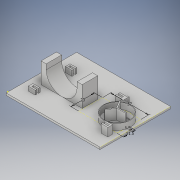
# Autodesk Inventor part: base
Saved by Autodesk Inventor 2019 (Build 230136000, 136)
## iProperties
Created: 2022-02-03
Part Number: base
Material: Generic
Document SubType Name: Modeling
Designer: josec
Density: 1 g/cm^3
Appearance: Default
Author: josec
Autodesk Inventor part; units mm, degrees
ref_plane "YZ Plane" through (0, 0, 0) normal (1, 0, 0) x (0, 1, 0)
ref_plane "XZ Plane" through (0, 0, 0) normal (0, 1, 0) x (-1, 0, 0)
ref_plane "XY Plane" through (0, 0, 0) normal (0, 0, 1) x (1, 0, 0)
sketch "Sketch1" plane through (0, 0, 0) normal (0, 1, 0) x (-1, 0, 0)
  line L0 (0, 0) -> (-90, 0)
  line L1 (-90, 0) -> (-90, -60)
  line L2 (-90, -60) -> (0, -60)
  line L3 (0, -60) -> (0, 0)
  dimension "d0" = 90
  dimension "d1" = 60
  constraints: 8 end point, 2 parallel, 1 horizontal, 1 perpendicular
  measures "d0" distance of L2.end L1.end
  measures "d1" distance of L1.end L0.end
extrude "Extrusion1" add sketch "Sketch1" along normal blind 2
sketch "Sketch2" plane through (0, 2, 0) normal (0, 1, 0) x (1, 0, 0)
  line L0 (90, 0) -> (90, 60) construction
  line L1 (90, 60) -> (85, 60) construction
  line L2 (90, 60) -> (0, 60) construction
  line L3 (85, 60) -> (85, 0) construction
  line L4 (0, 0) -> (90, 0) construction
  line L5 (85, 30) -> (85, 35.5) construction
  line L6 (85, 35.5) -> (85, 30) construction
  line L7 (85, 30) -> (85, 24.5) construction
  line L8 (85, 24.5) -> (79, 24.5)
  line L9 (79, 24.5) -> (79, 23.5)
  line L10 (79, 23.5) -> (85, 23.5)
  line L11 (85, 23.5) -> (85, 24.5)
  line L12 (85, 35.5) -> (79, 35.5)
  line L13 (79, 35.5) -> (79, 36.5)
  line L14 (79, 36.5) -> (85, 36.5)
  line L15 (85, 36.5) -> (85, 35.5)
  dimension "d4" = 5
  dimension "d5" = 5.5
  dimension "d6" = 5.5
  dimension "d7" = 6
  dimension "d8" = 1
  dimension "d9" = 1
  constraints: 26 end point, 4 parallel, 4 point on line, 2 horizontal, 2 perpendicular, 1 collinear, 1 midpoint, 1 vertical
  measures "d4" distance of L0.end L1.end
  measures "d5" distance of L5.start L5.end
  measures "d6" distance of L5.start L7.end
  measures "d7" distance of L10.end L9.end
  measures "d8" distance of L9.end L8.end
  measures "d9" distance of L12.end L13.end
extrude "Extrusion2" cut sketch "Sketch2" against normal through all
sketch "Sketch3" plane through (0, 2, 0) normal (0, 1, 0) x (1, 0, 0)
  line L0 (85, 35.5) -> (79, 35.5) construction
  line L1 (85, 24.5) -> (79, 24.5) construction
  line L2 (79, 35.5) -> (79, 24.5) construction
  line L3 (79, 30) -> (72.5, 30) construction
  line L4 (72.5, 30) -> (72.5, 32.5) construction
  line L5 (72.5, 32.5) -> (67.5, 32.5) construction
  line L6 (67.5, 32.5) -> (67.5, 27.5) construction
  line L7 (67.5, 27.5) -> (72.5, 27.5) construction
  line L8 (72.5, 27.5) -> (72.5, 32.5) construction
  line L9 (67.5, 27.5) -> (70.5, 27.5) construction
  line L10 (67.5, 32.5) -> (70.5, 32.5) construction
  arc A0 (70.5, 27.5) -> (70.5, 32.5) centre (69.9375, 30) ccw
  line L11 (70.5, 32.5) -> (67.5, 32.5) construction
  line L12 (67.5, 32.5) -> (67.5, 27.5) construction
  line L13 (67.5, 32.5) -> (70.5, 32.5)
  line L14 (67.5, 32.5) -> (67.5, 27.5)
  line L15 (67.5, 27.5) -> (70.5, 27.5)
  point P0 (0, 0)
  dimension "d12" = 6.5
  dimension "d15" = 2.5
  dimension "d16" = 5
  dimension "d17" = 5
  dimension "d18" = 3
  dimension "d19" = 3
  constraints: 28 end point, 4 perpendicular, 3 point on circle, 2 collinear, 2 horizontal, 2 parallel, 2 point on line, 2 vertical, 1 centre point, 1 midpoint
  measures "d12" distance of L3.start L3.end
  measures "d15" distance of L3.end L4.end
  measures "d16" distance of L7.end L6.end
  measures "d17" distance of L6.end L5.end
  measures "d18" distance of L6.end L9.end
  measures "d19" distance of L5.end L10.end
extrude "Extrusion3" cut sketch "Sketch3" against normal through all
sketch "Sketch5" plane through (0, 2, 0) normal (0, 1, 0) x (1, 0, 0)
  line L0 (85, 35.5) -> (85, 36.5) construction
  line L1 (85, 36.5) -> (67.5, 36.5) construction
  line L2 (67.5, 36.5) -> (67.5, 23.5) construction
  line L3 (67.5, 23.5) -> (85, 23.5) construction
  line L4 (85, 23.5) -> (85, 36.5) construction
  circle A0 centre (76.25, 30) radius 12.5 construction
  line L5 (76.25, 30) -> (85, 30) construction
  line L6 (85, 30) -> (85, 30.5) construction
  line L7 (85, 30.5) -> (76.25, 30.5)
  line L8 (76.25, 30.5) -> (76.25, 29.5)
  line L9 (76.25, 29.5) -> (85, 29.5)
  line L10 (85, 29.5) -> (85, 30.5)
  line L11 (76.25, 30) -> (71.875, 37.5777) construction
  line L12 (71.875, 37.5777) -> (71.442, 37.3277) construction
  line L13 (71.442, 37.3277) -> (75.817, 29.75)
  line L14 (75.817, 29.75) -> (76.683, 30.25)
  line L15 (76.683, 30.25) -> (72.308, 37.8277)
  line L16 (72.308, 37.8277) -> (71.442, 37.3277)
  line L17 (76.25, 30) -> (71.875, 22.4223) construction
  line L18 (71.875, 22.4223) -> (72.308, 22.1723) construction
  line L19 (72.308, 22.1723) -> (76.683, 29.75)
  line L20 (76.683, 29.75) -> (75.817, 30.25)
  line L21 (75.817, 30.25) -> (71.442, 22.6723)
  line L22 (71.442, 22.6723) -> (72.308, 22.1723)
  point P0 (0, 0)
  dimension "d32" = 13
  dimension "d33" = 25
  dimension "d34" = 0.5
  dimension "d35" = 1
  dimension "d38" = 360
  constraints: 44 end point, 4 parallel, 2 coincident, 2 horizontal, 2 perpendicular, 1 centre point, 1 midpoint, 1 point on line, 35 other
  measures "d32" distance of L2.end L1.end
  measures "d33" diameter of A0
  measures "d34" distance of L5.end L6.end
  measures "d35" distance of L8.end L7.end
extrude "Extrusion4" add sketch "Sketch5" along normal blind 10
sketch "Sketch6" plane through (0, 2, 0) normal (0, 1, 0) x (1, 0, 0)
  line L0 (85, 36.5) -> (85, 35.5) construction
  line L1 (85, 36.5) -> (67.5, 36.5) construction
  line L2 (67.5, 36.5) -> (67.5, 23.5) construction
  line L3 (67.5, 23.5) -> (85, 23.5) construction
  line L4 (85, 23.5) -> (85, 36.5) construction
  circle A0 centre (76.25, 30) radius 12.5
  circle A1 centre (76.25, 30) radius 13
  point P0 (0, 0)
  dimension "d42" = 13
  dimension "d43" = 25
  dimension "d44" = 26
  constraints: 8 end point, 2 centre point, 2 parallel, 1 coincident, 1 horizontal, 1 perpendicular
  measures "d42" distance of L2.end L1.end
  measures "d43" diameter of A0
  measures "d44" diameter of A1
extrude "Extrusion5" add sketch "Sketch6" along normal blind 6
sketch "Sketch7" plane through (0, 2, 0) normal (0, 1, 0) x (1, 0, 0)
  line L0 (90, 0) -> (90, 60) construction
  line L1 (90, 30) -> (90, 14) construction
  line L2 (90, 14) -> (0, 14) construction
  line L3 (0, 60) -> (0, 0) construction
  line L4 (90, 14) -> (85, 14) construction
  line L5 (85, 14) -> (11, 14) construction
  line L6 (11, 14) -> (11, 12.4) construction
  line L7 (11, 12.4) -> (85, 12.4) construction
  line L8 (85, 12.4) -> (85, 14) construction
  line L9 (85, 14) -> (85, 12.4)
  line L10 (85, 12.4) -> (80, 12.4)
  line L11 (85, 14) -> (80, 14)
  line L12 (80, 14) -> (80, 15.5)
  line L13 (80, 12.4) -> (80, 10.9)
  line L14 (11, 14) -> (16, 14)
  line L15 (16, 14) -> (16, 15.5)
  line L16 (16, 15.5) -> (9, 15.5)
  line L17 (11, 14) -> (11, 12.4)
  line L18 (11, 12.4) -> (16, 12.4)
  line L19 (16, 12.4) -> (16, 10.9)
  line L20 (16, 10.9) -> (9, 10.9)
  line L21 (9, 10.9) -> (9, 15.5)
  line L22 (80, 15.5) -> (86.5, 15.5)
  line L23 (80, 10.9) -> (86.5, 10.9)
  line L24 (86.5, 10.9) -> (86.5, 15.5)
  dimension "d47" = 16
  dimension "d48" = 5
  dimension "d49" = 74
  dimension "d50" = 1.6
  dimension "d51" = 5
  dimension "d52" = 5
  dimension "d53" = 1.5
  dimension "d55" = 1.5
  dimension "d57" = 5
  dimension "d58" = 1.5
  dimension "d59" = 7
  dimension "d60" = 5
  dimension "d61" = 1.5
  dimension "d62" = 6.5
  dimension "d63" = 6.5
  constraints: 46 end point, 8 perpendicular, 7 point on line, 3 horizontal, 3 vertical, 2 parallel, 1 midpoint
  measures "d47" distance of L1.start L1.end
  measures "d48" distance of L1.end L4.end
  measures "d49" distance of L7.end L6.end
  measures "d50" distance of L6.end L5.end
  measures "d51" distance of L7.end L10.end
  measures "d52" distance of L4.end L11.end
  measures "d53" distance of L11.end L12.end
  measures "d55" distance of L10.end L13.end
  measures "d57" distance of L5.end L14.end
  measures "d58" distance of L14.end L15.end
  measures "d59" distance of L15.end L16.end
  measures "d60" distance of L6.end L18.end
  measures "d61" distance of L18.end L19.end
  measures "d62" distance of L12.end L22.end
  measures "d63" distance of L13.end L23.end
extrude "Extrusion6" add sketch "Sketch7" along normal blind 4
sketch "Sketch8" plane through (0, 6, 0) normal (0, 1, 0) x (1, 0, 0)
  line L0 (80, 15.5) -> (80, 14) projected
  line L1 (80, 14) -> (80, 15.5)
  line L2 (86.5, 10.9) -> (86.5, 15.5) projected
  line L3 (80, 15.5) -> (86.5, 15.5)
  line L4 (86.5, 15.5) -> (86.5, 10.9)
  line L5 (80, 12.4) -> (80, 10.9) projected
  line L6 (86.5, 10.9) -> (80, 10.9)
  line L7 (80, 10.9) -> (80, 12.4)
  line L8 (85, 12.4) -> (80, 12.4) projected
  line L9 (80, 12.4) -> (85, 12.4)
  line L10 (85, 14) -> (85, 12.4) projected
  line L11 (85, 12.4) -> (85, 14)
  line L12 (80, 14) -> (85, 14) projected
  line L13 (85, 14) -> (80, 14)
  point P0 (0, 0)
  constraints: 16 end point, 4 perpendicular, 3 collinear, 1 vertical
extrude "Extrusion7" add sketch "Sketch8" along normal blind 4
sketch "Sketch10" plane through (0, 2, 0) normal (0, 1, 0) x (1, 0, 0)
  line L0 (90, 0) -> (90, 60) construction
  line L1 (90, 30) -> (50, 30) construction
  line L2 (50, 30) -> (50, 37.5) construction
  line L3 (50, 37.5) -> (10, 37.5)
  line L4 (10, 37.5) -> (10, 22.5)
  line L5 (10, 22.5) -> (50, 22.5)
  line L6 (50, 22.5) -> (50, 37.5)
  point P0 (0, 0)
  dimension "d82" = 40
  dimension "d83" = 7.5
  dimension "d84" = 40
  dimension "d85" = 15
  constraints: 12 end point, 2 horizontal, 2 parallel, 1 midpoint, 1 perpendicular, 1 vertical
  measures "d82" distance of L1.start L1.end
  measures "d83" distance of L1.end L2.end
  measures "d84" distance of L5.end L4.end
  measures "d85" distance of L4.end L3.end
extrude "Extrusion9" add sketch "Sketch10" along normal blind 15
sketch "Sketch11" plane through (10, 2, -22.5) normal (0, 0, 1) x (1, 0, 0)
  line L0 (0, 0) -> (0, 15) construction
  line L1 (0, 15) -> (20, 15) construction
  line L2 (40, 15) -> (0, 15) construction
  arc A0 (5, 15) -> (35, 15) centre (20, 15) ccw
  line L3 (5, 15) -> (35, 15)
  point P0 (-10, -2)
  dimension "d88" = 30
  constraints: 4 end point, 2 point on circle, 2 point on line, 1 centre point, 1 coincident, 1 collinear, 1 midpoint
  measures "d88" diameter of A0
extrude "Extrusion10" cut sketch "Sketch11" against normal blind 15
sketch "Sketch15" plane through (0, 2, 0) normal (0, 1, 0) x (1, 0, 0)
  line L0 (90, 0) -> (90, 60) construction
  line L1 (90, 30) -> (90, 45) construction
  line L2 (90, 45) -> (90, 45) construction
  line L3 (90, 45) -> (68, 45) construction
  line L4 (68, 45) -> (68, 65) construction
  line L5 (68, 65) -> (90, 65) construction
  line L6 (90, 65) -> (90, 45) construction
  line L7 (68, 45) -> (68, 50)
  line L8 (68, 50) -> (66.5, 50)
  line L9 (66.5, 50) -> (66.5, 45)
  line L10 (66.5, 45) -> (66.5, 43.5)
  line L11 (68, 45) -> (73, 45)
  line L12 (73, 45) -> (73, 43.5)
  line L13 (73, 43.5) -> (66.5, 43.5)
  line L14 (90, 60) -> (0, 60) projected
  point P0 (0, 0)
  dimension "d99" = 15
  dimension "d100" = 0
  dimension "d101" = 22
  dimension "d102" = 20
  dimension "d103" = 5
  dimension "d104" = 1.5
  dimension "d105" = 5
  dimension "d106" = 1.5
  constraints: 26 end point, 5 perpendicular, 4 point on line, 2 horizontal, 2 parallel, 1 midpoint
  measures "d99" distance of L1.start L1.end
  measures "d100" distance of L1.end L2.end
  measures "d101" distance of L4.end L5.end
  measures "d102" distance of L3.end L4.end
  measures "d103" distance of L3.end L7.end
  measures "d104" distance of L7.end L8.end
  measures "d105" distance of L3.end L11.end
  measures "d106" distance of L11.end L12.end
extrude "Extrusion13" add sketch "Sketch15" along normal blind 5
sketch "Sketch17" plane through (0, 17, 0) normal (0, 1, 0) x (1, 0, 0)
  line L0 (50, 37.5) -> (45, 37.5) projected
  line L1 (45, 22.5) -> (30, 22.5) projected
  line L2 (50, 37.5) -> (45, 37.5)
  line L3 (45, 37.5) -> (45, 22.5)
  line L4 (45, 22.5) -> (50, 22.5)
  line L5 (50, 22.5) -> (50, 37.5)
  line L6 (15, 37.5) -> (30, 37.5) projected
  line L7 (30, 22.5) -> (10, 22.5) projected
  line L8 (15, 37.5) -> (10, 37.5)
  line L9 (10, 37.5) -> (10, 22.5)
  line L10 (10, 22.5) -> (15, 22.5)
  line L11 (15, 22.5) -> (15, 37.5)
  point P0 (0, 0)
  constraints: 16 end point, 4 parallel, 2 horizontal, 2 perpendicular
extrude "Extrusion14" add sketch "Sketch17" along normal blind 5
sketch "Sketch18" plane through (0, 2, 0) normal (0, 1, 0) x (1, 0, 0)
  line L0 (90, 0) -> (90, 60) construction
  line L1 (90, 30) -> (90, 46) construction
  line L2 (90, 46) -> (0, 46) construction
  line L3 (66.5, 43.5) -> (66.5, 50) construction
  line L4 (66.5, 46) -> (65, 46) construction
  line L5 (65, 46) -> (13, 46) construction
  line L6 (13, 46) -> (13, 47.6) construction
  line L7 (13, 47.6) -> (65, 47.6) construction
  line L8 (65, 47.6) -> (65, 46) construction
  line L9 (65, 46) -> (60, 46)
  line L10 (60, 46) -> (60, 44.5)
  line L11 (60, 44.5) -> (66.5, 44.5)
  line L12 (65, 46) -> (65, 47.6)
  line L13 (65, 47.6) -> (60, 47.6)
  line L14 (60, 47.6) -> (60, 49.1)
  line L15 (60, 49.1) -> (66.5, 49.1)
  line L16 (66.5, 49.1) -> (66.5, 44.5)
  line L17 (13, 47.6) -> (13, 46)
  line L18 (13, 46) -> (18, 46)
  line L19 (18, 46) -> (18, 44.5)
  line L20 (18, 44.5) -> (11.5, 44.5)
  line L21 (13, 47.6) -> (18, 47.6)
  line L22 (18, 47.6) -> (18, 49.1)
  line L23 (18, 49.1) -> (11.5, 49.1)
  line L24 (11.5, 49.1) -> (11.5, 44.5)
  point P0 (0, 0)
  dimension "d115" = 16
  dimension "d116" = 1.5
  dimension "d117" = 52
  dimension "d118" = 1.6
  dimension "d119" = 5
  dimension "d120" = 1.5
  dimension "d121" = 5
  dimension "d122" = 1.5
  dimension "d123" = 5
  dimension "d124" = 1.5
  dimension "d125" = 6.5
  dimension "d126" = 1.5
  constraints: 46 end point, 11 perpendicular, 10 point on line, 2 collinear, 2 horizontal, 2 parallel, 1 midpoint
  measures "d115" distance of L1.start L1.end
  measures "d116" distance of L4.start L4.end
  measures "d117" distance of L6.end L7.end
  measures "d118" distance of L5.end L6.end
  measures "d119" distance of L4.end L9.end
  measures "d120" distance of L9.end L10.end
  measures "d121" distance of L7.end L13.end
  measures "d122" distance of L13.end L14.end
  measures "d123" distance of L5.end L18.end
  measures "d124" distance of L18.end L19.end
  measures "d125" distance of L19.end L20.end
  measures "d126" distance of L21.end L22.end
extrude "Extrusion15" add sketch "Sketch18" along normal blind 5
sketch "Sketch19" plane through (0, 0, 0) normal (0, 0, 1) x (1, 0, 0)
  line L0 (90, 2) -> (0, 2) projected
  line L1 (90, 0) -> (0, 0) projected
  line L2 (0, 2) -> (90, 2)
  line L3 (90, 2) -> (90, 0)
  line L4 (90, 0) -> (0, 0)
  line L5 (0, 0) -> (0, 2)
  constraints: 8 end point, 2 parallel, 1 horizontal, 1 perpendicular
extrude "Extrusion16" add sketch "Sketch19" along normal blind 1.5
sketch "Sketch20" plane through (90, 0, -60) normal (1, 0, 0) x (0, 0, -1)
  line L0 (0, 0) -> (0, 2) projected
  line L1 (0, 2) -> (-61.5, 2) projected
  line L2 (0, 0) -> (-61.5, 0)
  line L3 (-61.5, 0) -> (-61.5, 2)
  line L4 (-61.5, 2) -> (0, 2)
  line L5 (0, 2) -> (0, 0)
  point P0 (-60, 0)
  constraints: 8 end point, 2 parallel, 1 horizontal, 1 perpendicular
extrude "Extrusion17" add sketch "Sketch20" along normal blind 1.25
sketch "Sketch21" plane through (0, 0, -60) normal (0, 0, -1) x (-1, 0, 0)
  line L0 (0, 0) -> (-91.25, 0)
  line L1 (-91.25, 0) -> (-91.25, 2)
  line L2 (-91.25, 2) -> (0, 2)
  line L3 (0, 2) -> (0, 0)
  constraints: 8 end point, 2 parallel, 1 horizontal, 1 perpendicular
extrude "Extrusion18" add sketch "Sketch21" along normal blind 7
sketch "Sketch22" plane through (0, 2, 0) normal (0, 1, 0) x (1, 0, 0)
  line L0 (85, 30.5) -> (85, 29.5) construction
  line L1 (91.25, -1.5) -> (91.25, 67) construction
  line L2 (91.25, 30) -> (89.25, 30) construction
  line L3 (89.25, 30) -> (87.75, 30) construction
  line L4 (87.75, 30) -> (87.75, 18.5) construction
  line L5 (87.75, 18.5) -> (50.75, 18.5) construction
  line L6 (50.75, 18.5) -> (50.75, 41.5) construction
  line L7 (50.75, 41.5) -> (87.75, 41.5) construction
  line L8 (87.75, 41.5) -> (87.75, 18.5) construction
  point P0 (0, 0)
  dimension "d135" = 2
  dimension "d136" = 1.5
  dimension "d137" = 11.5
  dimension "d138" = 37
  dimension "d139" = 23
  constraints: 14 end point, 2 horizontal, 2 parallel, 1 perpendicular, 1 point on line, 1 vertical
  measures "d135" distance of L2.start L2.end
  measures "d136" distance of L2.end L3.end
  measures "d137" distance of L3.end L4.end
  measures "d138" distance of L6.end L7.end
  measures "d139" distance of L5.end L6.end
body "Solid1"
